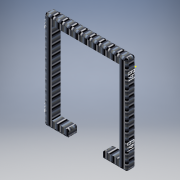
# Autodesk Inventor part: Bumpers
Saved by Autodesk Inventor 2017 (Build 210142000, 142)
## iProperties
Created: 2017-12-29
Part Number: Bumpers
Material: Fabric
Document SubType Name: Modeling
Designer: anikasoojin
Density: 0.9 g/cm^3
Appearance: Stripes - Black-White-Blue-Gray 1
Mass: 17846.8 g
Surface Area: 9464.7 cm^2
Volume: 19829.8 cm^3
Author: anikasoojin
Autodesk Inventor part; units mm, degrees
ref_plane "YZ Plane" through (0, 0, 0) normal (1, 0, 0) x (0, 1, 0)
ref_plane "XZ Plane" through (0, 0, 0) normal (0, 1, 0) x (-1, 0, 0)
ref_plane "XY Plane" through (0, 0, 0) normal (0, 0, 1) x (1, 0, 0)
sketch "Sketch1" plane through (0, 0, 0) normal (0, 0, 1) x (1, 0, 0)
  line L0 (0, 26.1238) -> (688.34, 26.1238)
  line L1 (688.34, 26.1238) -> (688.34, -814.6162)
  line L2 (0, 26.1238) -> (0, -814.6162)
  line L3 (0, -814.6162) -> (167.64, -814.6162)
  line L4 (688.34, -814.6162) -> (520.7, -814.6162)
  line L5 (520.7, -890.8162) -> (764.54, -890.8162)
  line L6 (764.54, -890.8162) -> (764.54, 102.3238)
  line L7 (764.54, 102.3238) -> (-76.2, 102.3238)
  line L8 (-76.2, 102.3238) -> (-76.2, -890.8162)
  line L9 (-76.2, -890.8162) -> (167.64, -890.8162)
  line L10 (167.64, -814.6162) -> (167.64, -890.8162)
  line L11 (520.7, -814.6162) -> (520.7, -890.8162)
  point P0 (0, 0)
  dimension "d0" = 688.34
  dimension "d1" = 840.74
  dimension "d2" = 167.64
  dimension "d3" = 167.64
  dimension "d4" = 76.2
  constraints: 24 end point, 4 vertical, 3 horizontal, 4 other
  measures "d0" distance of L0.start L0.end
  measures "d1" distance of L0.end L1.end
  measures "d2" distance of L2.end L3.end
  measures "d3" distance of L1.end L4.end
  measures "d4" distance between parallel lines of L1 L6
extrude "Extrusion1" add sketch "Sketch1" along normal blind 88.9
fillet "Fillet1" radius 19.05 18 edges at (-76.2, -394.2462, 88.9) (45.72, -890.8162, 88.9) (45.72, -890.8162, 0) (-76.2, -394.2462, 0) (-76.2, -890.8162, 44.45) (167.64, -890.8162, 44.45) (520.7, -890.8162, 44.45) (764.54, -890.8162, 44.45) (642.62, -890.8162, 88.9) (642.62, -890.8162, 0) (764.54, -394.2462, 88.9) (764.54, -394.2462, 0) (764.54, 102.3238, 44.45) (344.17, 102.3238, 88.9) (344.17, 102.3238, 0) (-76.2, 102.3238, 44.45) (520.7, -814.6162, 44.45) (167.64, -814.6162, 44.45)
sketch "Sketch2" plane through (764.54, -871.7662, 19.05) normal (1, 0, 0) x (0, 0, -1)
  line L0 (-65.2441, 154.6268) -> (-65.2441, 182.3935) construction
  line L1 (-65.2441, 182.3935) -> (47.3065, 182.3935) construction
  line L2 (47.3065, 182.3935) -> (47.3065, 154.6268) construction
  line L3 (47.3065, 154.6268) -> (-65.2441, 154.6268) construction
  line L4 (-58.9935, 771.5963) -> (-58.9935, 799.363) construction
  line L5 (-58.9935, 799.363) -> (53.557, 799.363) construction
  line L6 (53.557, 799.363) -> (53.557, 771.5963) construction
  line L7 (53.557, 771.5963) -> (-58.9935, 771.5963) construction
  point P0 (19.05, 871.7662)
  dimension "d3" = 167.64
  constraints: 4 other
sketch "Sketch3" plane through (-76.2, -871.7662, 19.05) normal (-1, 0, 0) x (0, 0, 1)
  line L0 (66.8415, 917.1452) -> (66.8415, 824.847) construction
  line L1 (66.8415, 824.847) -> (-3.0085, 824.847) construction
  line L2 (-3.0085, 824.847) -> (-3.0085, 917.1452) construction
  line L3 (-3.0085, 917.1452) -> (66.8415, 917.1452) construction
  line L4 (68.429, 179.765) -> (68.429, 87.4668) construction
  line L5 (68.429, 87.4668) -> (-1.421, 87.4668) construction
  line L6 (-1.421, 87.4668) -> (-1.421, 179.765) construction
  line L7 (-1.421, 179.765) -> (68.429, 179.765) construction
  point P0 (-19.05, 871.7662)
  dimension "d3" = 167.64
  constraints: 4 other
body "Solid1"
